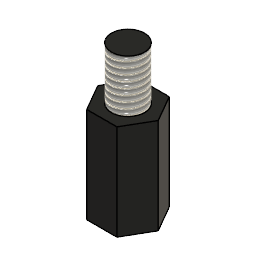
Standoff 7mm_v2 (Autodesk Fusion 360 design; units mm, degrees)
Autodesk Fusion 360 part; units mm, degrees
sketch "Sketch1" plane through (0, 0, 0) normal (0, 0, 1) x (1, 0, 0)
  circle A0 centre (0, 0) radius 1.25
  line L0 (2.3094, 0) -> (1.1547, 2)
  line L1 (1.1547, 2) -> (-1.1547, 2)
  line L2 (-1.1547, 2) -> (-2.3094, 0)
  line L3 (-2.3094, 0) -> (-1.1547, -2)
  line L4 (-1.1547, -2) -> (1.1547, -2)
  line L5 (1.1547, -2) -> (2.3094, 0)
  dimension "d1" = 2.5
  dimension "d21" = 2
  constraint coincident A0.centre origin
  constraint horizontal L1
  measures "d1" diameter of A0
  measures "d21" distance of A0.centre L4
extrude "Extrude6" add sketch "Sketch1" along normal blind 6
extrude "Extrude7" add sketch "Sketch1" along normal blind 5 from surface at 5 contours A0
thread "Thread1" "ISO Metric profile 2.6 M2.6x0.45 M2.6x0.45 6g" major diameter 2.53 minor diameter 2.0162 pitch 0.45 angle 60 resizes the face on face at (1.2438, -0.1245, 8.6667)
thread "Thread2" "ISO Metric profile 2.5 M2.5x0.45 M2.5x0.45 6H" major diameter 2.58 minor diameter 2.0755 pitch 0.45 angle 60 resizes the face on face at (1.2484, 0.0623, 1.6667)
move_face "OffsetFaces2" offset 1.3 1 faces at (-1.4664, 0.8168, 0)
